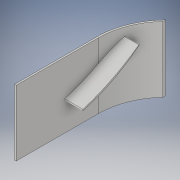
# Autodesk Inventor part: type8_end_plate
Saved by Autodesk Inventor 2018.1 (Build 221171000, 171)
## iProperties
Created: 2017-11-03
Part Number: type8_end_plate
Material: 一般
Document SubType Name: Modeling
Designer: ku_sk
Density: 1 g/cm^3
Appearance: 既定
Author: ku_sk
Autodesk Inventor part; units mm, degrees
ref_plane "YZ Plane" through (0, 0, 0) normal (1, 0, 0) x (0, 1, 0)
ref_plane "XZ Plane" through (0, 0, 0) normal (0, 1, 0) x (-1, 0, 0)
ref_plane "XY Plane" through (0, 0, 0) normal (0, 0, 1) x (1, 0, 0)
sketch "スケッチ1" plane through (0, 0, 0) normal (1, 0, 0) x (0, 1, 0)
  line L0 (100, 200) -> (-100, 200)
  line L1 (-100, 200) -> (-100, -200)
  line L2 (-100, -200) -> (100, -200)
  line L3 (100, -200) -> (100, 200)
  line L4 (-140, 0) -> (140, 0) projected
  line L5 (0, -280) -> (0, 280) projected
  point P0 (0, 0)
  point P1 (100, 0)
  point P2 (0, 200)
  dimension "d2" = 200
  dimension "d3" = 400
  constraints: 8 end point, 2 midpoint, 2 parallel, 2 point on line, 1 horizontal, 1 perpendicular
  measures "d2" distance of L1.end L2.end
  measures "d3" distance of L2.end L0.start
extrude "押し出し1" add sketch "スケッチ1" along normal mid plane 60
sketch "スケッチ3" plane through (-30, 100, 200) normal (0, 1, 0) x (1, 0, 0)
  line L0 (0, 0) -> (60, 0) projected
  line L1 (60, 0) -> (5, 0)
  line L2 (60, 392) -> (60, 0)
  line L3 (60, 400) -> (60, 0) projected
  line L4 (5, 0) -> (5, 250)
  arc A0 (60, 392) -> (5, 250) centre (215.8091, 250) ccw
  line L5 (0, 0) -> (0, 400) projected
  line L6 (0, 400) -> (60, 400) projected
  arc A1 (60, 400) -> (0, 264.2446) centre (215.8091, 250) ccw
  dimension "d16" = 5
  dimension "d18" = 250
  dimension "d21" = 8
  constraints: 6 end point, 4 point on circle, 2 centre point, 2 point on line, 1 collinear, 1 concentric, 1 horizontal, 1 tangent, 1 vertical
  measures "d16" distance between parallel lines of L5 L4
  measures "d18" distance of L1.end L4.end
  measures "d21" distance from line of L2.start L6
extrude "押し出し2" cut sketch "スケッチ3" against normal through all contours L4 A0 L2 L0 | L5 L6 A1
sketch "スケッチ7" plane through (-25, 100, 200) normal (1, 0, 0) x (0, 0, -1)
  arc A0 (50, -130) -> (350, 0) centre (-10.3611, 420.4486) ccw
  arc A1 (50, -130) -> (350, 0) centre (25.3027, 338.1476) ccw
  line L0 (50, -130) -> (350, 0)
  line L1 (0, -200) -> (0, 0) projected
  line L2 (0, 0) -> (250, 0) projected
  line L3 (400, -200) -> (400, 0) projected
  dimension "d30" = 50
  dimension "d31" = 130
  dimension "d38" = 50
  constraints: 4 point on circle, 2 centre point, 2 end point, 1 point on line
  measures "d30" distance from line of L1 L0.start
  measures "d31" distance from line of L2 L0.start
  measures "d38" distance from line of L3 L0.end
extrude "押し出し5" add sketch "スケッチ7" along normal blind 55 contours A0 A1
sketch "スケッチ8" plane through (0, 0, 0) normal (0, 1, 0) x (-1, 0, 0)
  line L0 (-30, -200) -> (-30, -192) projected
  line L1 (-30, -200) -> (30, -200)
  line L2 (30, 200) -> (30, -64.2446) projected
  arc A0 (-30, -200) -> (30, -64.2446) centre (-185.8091, -50) ccw projected
  arc A1 (-30, -200) -> (-30, -200) centre (-53.5814, -108.4409) ccw
  line L3 (30, -200) -> (30, -64.2446)
  point P0 (0, 0)
  constraints: 4 end point, 1 collinear, 1 horizontal, 4 other
extrude "押し出し6" cut sketch "スケッチ8" along normal through all contours A1 L3 L1 | A0 L3 A1
fillet "フィレット2" radius 1 1 edges at (15.1138, 100, -150)
fillet "フィレット2" radius 2 1 edges at (2.5, -30, 150)
